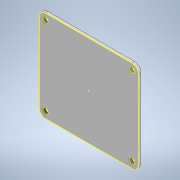
# Autodesk Inventor part: Controller_PCB
Saved by Autodesk Inventor 2021 (Build 250183000, 183)
## iProperties
Created: 2020-09-09
Part Number: Controller_PCB
Material: Generic
Document SubType Name: Modeling
Designer: Viktor
Density: 1 g/cm^3
Appearance: Default
Author: Viktor
Autodesk Inventor part; units mm, degrees
ref_plane "YZ Plane" through (0, 0, 0) normal (1, 0, 0) x (0, 1, 0)
ref_plane "XZ Plane" through (0, 0, 0) normal (0, 1, 0) x (-1, 0, 0)
ref_plane "XY Plane" through (0, 0, 0) normal (0, 0, 1) x (1, 0, 0)
sketch "Sketch1" plane through (0, 0, 0) normal (0, 0, 1) x (1, 0, 0)
  line L0 (-31, -28.5) -> (31, -28.5)
  line L1 (31, -28.5) -> (31, 28.5)
  line L2 (31, 28.5) -> (-31, 28.5)
  line L3 (-31, 28.5) -> (-31, -28.5)
  line L4 (-31, -28.5) -> (31, 28.5) construction
  line L5 (31, -28.5) -> (-31, 28.5) construction
  point P0 (0, 0)
  dimension "d0" = 62
  dimension "d1" = 57
  constraints: 12 end point, 2 midpoint, 2 parallel, 1 horizontal, 1 perpendicular
  measures "d0" distance of L1.end L2.end
  measures "d1" distance of L2.end L0.start
extrude "Extrusion1" add sketch "Sketch1" along normal blind 1.6
fillet "Fillet1" radius 4 4 edges at (31, 28.5, 0.8) (-31, 28.5, 0.8) (-31, -28.5, 0.8) (31, -28.5, 0.8)
sketch "Sketch2" plane through (0, 0, 1.6) normal (0, 0, 1) x (1, 0, 0)
  circle A0 centre (-27, 24.5) radius 1.6
  line L0 (-43.4, 0) -> (43.4, 0) projected
  line L1 (0, -39.9) -> (0, 39.9) construction
  line L2 (-31, 24.5) -> (-31, -24.5) construction
  line L3 (27, 28.5) -> (-27, 28.5) construction
  circle A1 centre (27, 24.5) radius 1.6
  circle A2 centre (-27, -24.5) radius 1.6
  line L4 (27, -28.5) -> (-27, -28.5) construction
  circle A3 centre (27, -24.5) radius 1.6
  point P0 (0, 0)
  dimension "d5" = 4
  dimension "d6" = 4
  dimension "d7" = 3.2
  constraints: 5 symmetric about line, 4 centre point, 2 end point, 3 other
  measures "d5" distance from line of L2 A0.centre
  measures "d6" distance from line of L3 A0.centre
  measures "d7" diameter of A0
extrude "Extrusion2" cut sketch "Sketch2" against normal through all
sketch "Sketch3" plane through (0, 0, 1.6) normal (0, 0, 1) x (1, 0, 0)
  circle A0 centre (-27, -24.5) radius 1.6 projected
  circle A1 centre (27, 24.5) radius 1.6 projected
  circle A2 centre (27, -24.5) radius 1.6 projected
  circle A3 centre (-27, 24.5) radius 1.6 projected
  arc A4 (27, -28.5) -> (31, -24.5) centre (27, -24.5) ccw projected
  line L0 (31, -24.5) -> (31, 24.5) projected
  arc A5 (31, 24.5) -> (27, 28.5) centre (27, 24.5) ccw projected
  line L1 (27, 28.5) -> (-27, 28.5) projected
  arc A6 (-27, 28.5) -> (-31, 24.5) centre (-27, 24.5) ccw projected
  line L2 (-31, 24.5) -> (-31, -24.5) projected
  arc A7 (-31, -24.5) -> (-27, -28.5) centre (-27, -24.5) ccw projected
  line L3 (-27, -28.5) -> (27, -28.5) projected
  point P0 (0, 0)
equation "\"d6\" = d5"
body "Solid1"
